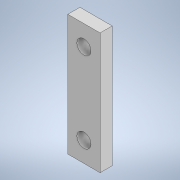
# Autodesk Inventor part: 3SR14_ポテンショメータ固定台
Saved by Autodesk Inventor 2021 (Build 250183000, 183)
## iProperties
Created: 2021-04-24
Part Number: 3SR14_ポテンショメータ固定台
Material: 一般
Document SubType Name: Modeling
Designer: ryusei
Density: 1 g/cm^3
Appearance: 既定
Author: ryusei
Autodesk Inventor part; units mm, degrees
ref_plane "YZ Plane" through (0, 0, 0) normal (1, 0, 0) x (0, 1, 0)
ref_plane "XZ Plane" through (0, 0, 0) normal (0, 1, 0) x (-1, 0, 0)
ref_plane "XY Plane" through (0, 0, 0) normal (0, 0, 1) x (1, 0, 0)
sketch "スケッチ1" plane through (0, 0, 0) normal (0, 0, 1) x (1, 0, 0)
  line L0 (0, 0) -> (8, 0)
  line L1 (8, 0) -> (8, 30)
  line L2 (8, 30) -> (0, 30)
  line L3 (0, 30) -> (0, 0)
  dimension "d0" = 8
  dimension "d1" = 30
  constraints: 8 end point, 2 parallel, 1 horizontal, 1 perpendicular
  measures "d0" distance between parallel lines of L1 L3
  measures "d1" distance between parallel lines of L0 L2
extrude "押し出し1" add sketch "スケッチ1" along normal blind 3
sketch "スケッチ2" plane through (0, 0, 3) normal (0, 0, 1) x (1, 0, 0)
  line L0 (8, 0) -> (8, 30) projected
  line L1 (8, 30) -> (0, 30) projected
  line L2 (0, 0) -> (8, 0) projected
  point P0 (4, 25)
  point P1 (4, 5)
  dimension "d4" = 4
  dimension "d5" = 5
  dimension "d6" = 5
  dimension "d7" = 4
  measures "d4" distance from line of L0 point (4, 25)
  measures "d5" distance from line of point (4, 25) L1
  measures "d6" distance from line of L2 point (4, 5)
  measures "d7" distance from line of L0 point (4, 5)
hole "穴1" at (4, 25, 3) at (4, 5, 3) direction (0, 0, -1) diameter 3.5 end through all
